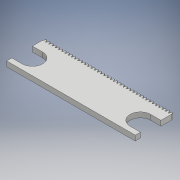
# Autodesk Inventor part: RescueKit-Slidev2
Saved by Autodesk Inventor 2018.3 (Build 223284000, 284)
## iProperties
Created: 2019-03-13
Part Number: RescueKit-Slidev2
Material: 一般
Document SubType Name: Modeling
Designer: shun2
Density: 1 g/cm^3
Appearance: 既定
Author: shun2
Autodesk Inventor part; units mm, degrees
ref_plane "YZ Plane" through (0, 0, 0) normal (1, 0, 0) x (0, 1, 0)
ref_plane "XZ Plane" through (0, 0, 0) normal (0, 1, 0) x (-1, 0, 0)
ref_plane "XY Plane" through (0, 0, 0) normal (0, 0, 1) x (1, 0, 0)
sketch "スケッチ1" plane through (0, 0, 0) normal (0, 0, 1) x (1, 0, 0)
  line L0 (125, 35.6665) -> (124.5146, 37)
  line L1 (124.5146, 37) -> (123.6718, 37)
  line L2 (123.6718, 37) -> (122.9438, 35)
  arc A0 (122.5868, 34.75) -> (122.9438, 35) centre (122.5868, 35.13) ccw
  line L3 (122.5868, 34.75) -> (122.458, 34.75)
  arc A1 (122.101, 35) -> (122.458, 34.75) centre (122.458, 35.13) ccw
  line L4 (122.101, 35) -> (121.373, 37)
  line L5 (121.373, 37) -> (120.5302, 37)
  line L6 (120.5302, 37) -> (119.8022, 35)
  arc A2 (119.4452, 34.75) -> (119.8022, 35) centre (119.4452, 35.13) ccw
  line L7 (119.4452, 34.75) -> (119.3164, 34.75)
  arc A3 (118.9594, 35) -> (119.3164, 34.75) centre (119.3164, 35.13) ccw
  line L8 (118.9594, 35) -> (118.2314, 37)
  line L9 (118.2314, 37) -> (117.3886, 37)
  line L10 (117.3886, 37) -> (116.6606, 35)
  arc A4 (116.3036, 34.75) -> (116.6606, 35) centre (116.3036, 35.13) ccw
  line L11 (116.3036, 34.75) -> (116.1748, 34.75)
  arc A5 (115.8178, 35) -> (116.1748, 34.75) centre (116.1748, 35.13) ccw
  line L12 (115.8178, 35) -> (115.0898, 37)
  line L13 (115.0898, 37) -> (114.247, 37)
  line L14 (114.247, 37) -> (113.519, 35)
  arc A6 (113.162, 34.75) -> (113.519, 35) centre (113.162, 35.13) ccw
  line L15 (113.162, 34.75) -> (113.0332, 34.75)
  arc A7 (112.6762, 35) -> (113.0332, 34.75) centre (113.0332, 35.13) ccw
  line L16 (112.6762, 35) -> (111.9482, 37)
  line L17 (111.9482, 37) -> (111.1054, 37)
  line L18 (111.1054, 37) -> (110.3774, 35)
  arc A8 (110.0204, 34.75) -> (110.3774, 35) centre (110.0204, 35.13) ccw
  line L19 (110.0204, 34.75) -> (109.8916, 34.75)
  arc A9 (109.5346, 35) -> (109.8916, 34.75) centre (109.8916, 35.13) ccw
  line L20 (109.5346, 35) -> (108.8066, 37)
  line L21 (108.8066, 37) -> (107.9638, 37)
  line L22 (107.9638, 37) -> (107.2358, 35)
  arc A10 (106.8788, 34.75) -> (107.2358, 35) centre (106.8788, 35.13) ccw
  line L23 (106.8788, 34.75) -> (106.75, 34.75)
  arc A11 (106.393, 35) -> (106.75, 34.75) centre (106.75, 35.13) ccw
  line L24 (106.393, 35) -> (105.665, 37)
  line L25 (105.665, 37) -> (104.8222, 37)
  line L26 (104.8222, 37) -> (104.0942, 35)
  arc A12 (103.7372, 34.75) -> (104.0942, 35) centre (103.7372, 35.13) ccw
  line L27 (103.7372, 34.75) -> (103.6084, 34.75)
  arc A13 (103.2514, 35) -> (103.6084, 34.75) centre (103.6084, 35.13) ccw
  line L28 (103.2514, 35) -> (102.5234, 37)
  line L29 (102.5234, 37) -> (101.6806, 37)
  line L30 (101.6806, 37) -> (100.9526, 35)
  arc A14 (100.5956, 34.75) -> (100.9526, 35) centre (100.5956, 35.13) ccw
  line L31 (100.5956, 34.75) -> (100.4668, 34.75)
  arc A15 (100.1098, 35) -> (100.4668, 34.75) centre (100.4668, 35.13) ccw
  line L32 (100.1098, 35) -> (99.3818, 37)
  line L33 (99.3818, 37) -> (98.539, 37)
  line L34 (98.539, 37) -> (97.811, 35)
  arc A16 (97.454, 34.75) -> (97.811, 35) centre (97.454, 35.13) ccw
  line L35 (97.454, 34.75) -> (97.3252, 34.75)
  arc A17 (96.9682, 35) -> (97.3252, 34.75) centre (97.3252, 35.13) ccw
  line L36 (96.9682, 35) -> (96.2402, 37)
  line L37 (96.2402, 37) -> (95.3974, 37)
  line L38 (95.3974, 37) -> (94.6694, 35)
  arc A18 (94.3124, 34.75) -> (94.6694, 35) centre (94.3124, 35.13) ccw
  line L39 (94.3124, 34.75) -> (94.1836, 34.75)
  arc A19 (93.8266, 35) -> (94.1836, 34.75) centre (94.1836, 35.13) ccw
  line L40 (93.8266, 35) -> (93.0986, 37)
  line L41 (93.0986, 37) -> (92.2558, 37)
  line L42 (92.2558, 37) -> (91.5278, 35)
  arc A20 (91.1708, 34.75) -> (91.5278, 35) centre (91.1708, 35.13) ccw
  line L43 (91.1708, 34.75) -> (91.042, 34.75)
  arc A21 (90.685, 35) -> (91.042, 34.75) centre (91.042, 35.13) ccw
  line L44 (90.685, 35) -> (89.957, 37)
  line L45 (89.957, 37) -> (89.1142, 37)
  line L46 (89.1142, 37) -> (88.3862, 35)
  arc A22 (88.0292, 34.75) -> (88.3862, 35) centre (88.0292, 35.13) ccw
  line L47 (88.0292, 34.75) -> (87.9004, 34.75)
  arc A23 (87.5434, 35) -> (87.9004, 34.75) centre (87.9004, 35.13) ccw
  line L48 (87.5434, 35) -> (86.8154, 37)
  line L49 (86.8154, 37) -> (85.9726, 37)
  line L50 (85.9726, 37) -> (85.2446, 35)
  arc A24 (84.8876, 34.75) -> (85.2446, 35) centre (84.8876, 35.13) ccw
  line L51 (84.8876, 34.75) -> (84.7588, 34.75)
  arc A25 (84.4018, 35) -> (84.7588, 34.75) centre (84.7588, 35.13) ccw
  line L52 (84.4018, 35) -> (83.6738, 37)
  line L53 (83.6738, 37) -> (82.831, 37)
  line L54 (82.831, 37) -> (82.103, 35)
  arc A26 (81.746, 34.75) -> (82.103, 35) centre (81.746, 35.13) ccw
  line L55 (81.746, 34.75) -> (81.6172, 34.75)
  arc A27 (81.2602, 35) -> (81.6172, 34.75) centre (81.6172, 35.13) ccw
  line L56 (81.2602, 35) -> (80.5322, 37)
  line L57 (80.5322, 37) -> (79.6894, 37)
  line L58 (79.6894, 37) -> (78.9614, 35)
  arc A28 (78.6044, 34.75) -> (78.9614, 35) centre (78.6044, 35.13) ccw
  line L59 (78.6044, 34.75) -> (78.4756, 34.75)
  arc A29 (78.1186, 35) -> (78.4756, 34.75) centre (78.4756, 35.13) ccw
  line L60 (78.1186, 35) -> (77.3906, 37)
  line L61 (77.3906, 37) -> (76.5478, 37)
  line L62 (76.5478, 37) -> (75.8198, 35)
  arc A30 (75.4628, 34.75) -> (75.8198, 35) centre (75.4628, 35.13) ccw
  line L63 (75.4628, 34.75) -> (75.334, 34.75)
  arc A31 (74.977, 35) -> (75.334, 34.75) centre (75.334, 35.13) ccw
  line L64 (74.977, 35) -> (74.249, 37)
  line L65 (74.249, 37) -> (73.4062, 37)
  line L66 (73.4062, 37) -> (72.6782, 35)
  arc A32 (72.3212, 34.75) -> (72.6782, 35) centre (72.3212, 35.13) ccw
  line L67 (72.3212, 34.75) -> (72.1924, 34.75)
  arc A33 (71.8354, 35) -> (72.1924, 34.75) centre (72.1924, 35.13) ccw
  line L68 (71.8354, 35) -> (71.1074, 37)
  line L69 (71.1074, 37) -> (70.2646, 37)
  line L70 (70.2646, 37) -> (69.5366, 35)
  arc A34 (69.1796, 34.75) -> (69.5366, 35) centre (69.1796, 35.13) ccw
  line L71 (69.1796, 34.75) -> (69.0508, 34.75)
  arc A35 (68.6938, 35) -> (69.0508, 34.75) centre (69.0508, 35.13) ccw
  line L72 (68.6938, 35) -> (67.9658, 37)
  line L73 (67.9658, 37) -> (67.123, 37)
  line L74 (67.123, 37) -> (66.395, 35)
  arc A36 (66.038, 34.75) -> (66.395, 35) centre (66.038, 35.13) ccw
  line L75 (66.038, 34.75) -> (65.9092, 34.75)
  arc A37 (65.5522, 35) -> (65.9092, 34.75) centre (65.9092, 35.13) ccw
  line L76 (65.5522, 35) -> (64.8242, 37)
  line L77 (64.8242, 37) -> (63.9814, 37)
  line L78 (63.9814, 37) -> (63.2534, 35)
  arc A38 (62.8964, 34.75) -> (63.2534, 35) centre (62.8964, 35.13) ccw
  line L79 (62.8964, 34.75) -> (62.7676, 34.75)
  arc A39 (62.4106, 35) -> (62.7676, 34.75) centre (62.7676, 35.13) ccw
  line L80 (62.4106, 35) -> (61.6826, 37)
  line L81 (61.6826, 37) -> (60.8398, 37)
  line L82 (60.8398, 37) -> (60.1118, 35)
  arc A40 (59.7548, 34.75) -> (60.1118, 35) centre (59.7548, 35.13) ccw
  line L83 (59.7548, 34.75) -> (59.626, 34.75)
  arc A41 (59.269, 35) -> (59.626, 34.75) centre (59.626, 35.13) ccw
  line L84 (59.269, 35) -> (58.541, 37)
  line L85 (58.541, 37) -> (57.6982, 37)
  line L86 (57.6982, 37) -> (56.9702, 35)
  arc A42 (56.6132, 34.75) -> (56.9702, 35) centre (56.6132, 35.13) ccw
  line L87 (56.6132, 34.75) -> (56.4844, 34.75)
  arc A43 (56.1274, 35) -> (56.4844, 34.75) centre (56.4844, 35.13) ccw
  line L88 (56.1274, 35) -> (55.3994, 37)
  line L89 (55.3994, 37) -> (54.5566, 37)
  line L90 (54.5566, 37) -> (53.8286, 35)
  arc A44 (53.4716, 34.75) -> (53.8286, 35) centre (53.4716, 35.13) ccw
  line L91 (53.4716, 34.75) -> (53.3428, 34.75)
  arc A45 (52.9858, 35) -> (53.3428, 34.75) centre (53.3428, 35.13) ccw
  line L92 (52.9858, 35) -> (52.2578, 37)
  line L93 (52.2578, 37) -> (51.415, 37)
  line L94 (51.415, 37) -> (50.687, 35)
  arc A46 (50.33, 34.75) -> (50.687, 35) centre (50.33, 35.13) ccw
  line L95 (50.33, 34.75) -> (50.2012, 34.75)
  arc A47 (49.8442, 35) -> (50.2012, 34.75) centre (50.2012, 35.13) ccw
  line L96 (49.8442, 35) -> (49.1162, 37)
  line L97 (49.1162, 37) -> (48.2734, 37)
  line L98 (48.2734, 37) -> (47.5454, 35)
  arc A48 (47.1884, 34.75) -> (47.5454, 35) centre (47.1884, 35.13) ccw
  line L99 (47.1884, 34.75) -> (47.0596, 34.75)
  arc A49 (46.7026, 35) -> (47.0596, 34.75) centre (47.0596, 35.13) ccw
  line L100 (46.7026, 35) -> (45.9746, 37)
  line L101 (45.9746, 37) -> (45.1318, 37)
  line L102 (45.1318, 37) -> (44.4038, 35)
  arc A50 (44.0468, 34.75) -> (44.4038, 35) centre (44.0468, 35.13) ccw
  line L103 (44.0468, 34.75) -> (43.918, 34.75)
  arc A51 (43.561, 35) -> (43.918, 34.75) centre (43.918, 35.13) ccw
  line L104 (43.561, 35) -> (42.833, 37)
  line L105 (42.833, 37) -> (41.9902, 37)
  line L106 (41.9902, 37) -> (41.2622, 35)
  arc A52 (40.9052, 34.75) -> (41.2622, 35) centre (40.9052, 35.13) ccw
  line L107 (40.9052, 34.75) -> (40.7764, 34.75)
  arc A53 (40.4194, 35) -> (40.7764, 34.75) centre (40.7764, 35.13) ccw
  line L108 (40.4194, 35) -> (39.6914, 37)
  line L109 (39.6914, 37) -> (38.8486, 37)
  line L110 (38.8486, 37) -> (38.1206, 35)
  arc A54 (37.7636, 34.75) -> (38.1206, 35) centre (37.7636, 35.13) ccw
  line L111 (37.7636, 34.75) -> (37.6348, 34.75)
  arc A55 (37.2778, 35) -> (37.6348, 34.75) centre (37.6348, 35.13) ccw
  line L112 (37.2778, 35) -> (36.5498, 37)
  line L113 (36.5498, 37) -> (35.707, 37)
  line L114 (35.707, 37) -> (34.979, 35)
  arc A56 (34.622, 34.75) -> (34.979, 35) centre (34.622, 35.13) ccw
  line L115 (34.622, 34.75) -> (34.4932, 34.75)
  arc A57 (34.1362, 35) -> (34.4932, 34.75) centre (34.4932, 35.13) ccw
  line L116 (34.1362, 35) -> (33.4082, 37)
  line L117 (33.4082, 37) -> (32.5654, 37)
  line L118 (32.5654, 37) -> (31.8374, 35)
  arc A58 (31.4804, 34.75) -> (31.8374, 35) centre (31.4804, 35.13) ccw
  line L119 (31.4804, 34.75) -> (31.3516, 34.75)
  arc A59 (30.9946, 35) -> (31.3516, 34.75) centre (31.3516, 35.13) ccw
  line L120 (30.9946, 35) -> (30.2666, 37)
  line L121 (30.2666, 37) -> (29.4238, 37)
  line L122 (29.4238, 37) -> (28.6958, 35)
  arc A60 (28.3388, 34.75) -> (28.6958, 35) centre (28.3388, 35.13) ccw
  line L123 (28.3388, 34.75) -> (28.21, 34.75)
  arc A61 (27.853, 35) -> (28.21, 34.75) centre (28.21, 35.13) ccw
  line L124 (27.853, 35) -> (27.125, 37)
  line L125 (27.125, 37) -> (26.2822, 37)
  line L126 (26.2822, 37) -> (25.5542, 35)
  arc A62 (25.1972, 34.75) -> (25.5542, 35) centre (25.1972, 35.13) ccw
  line L127 (25.1972, 34.75) -> (25.0684, 34.75)
  arc A63 (24.7114, 35) -> (25.0684, 34.75) centre (25.0684, 35.13) ccw
  line L128 (24.7114, 35) -> (23.9834, 37)
  line L129 (23.9834, 37) -> (23.1406, 37)
  line L130 (23.1406, 37) -> (22.4126, 35)
  arc A64 (22.0556, 34.75) -> (22.4126, 35) centre (22.0556, 35.13) ccw
  line L131 (22.0556, 34.75) -> (21.9268, 34.75)
  arc A65 (21.5698, 35) -> (21.9268, 34.75) centre (21.9268, 35.13) ccw
  line L132 (21.5698, 35) -> (20.8418, 37)
  line L133 (20.8418, 37) -> (19.999, 37)
  line L134 (19.999, 37) -> (19.271, 35)
  arc A66 (18.914, 34.75) -> (19.271, 35) centre (18.914, 35.13) ccw
  line L135 (18.914, 34.75) -> (18.7852, 34.75)
  arc A67 (18.4282, 35) -> (18.7852, 34.75) centre (18.7852, 35.13) ccw
  line L136 (18.4282, 35) -> (17.7002, 37)
  line L137 (17.7002, 37) -> (16.8574, 37)
  line L138 (16.8574, 37) -> (16.1294, 35)
  arc A68 (15.7724, 34.75) -> (16.1294, 35) centre (15.7724, 35.13) ccw
  line L139 (15.7724, 34.75) -> (15.6436, 34.75)
  arc A69 (15.2866, 35) -> (15.6436, 34.75) centre (15.6436, 35.13) ccw
  line L140 (15.2866, 35) -> (14.5586, 37)
  line L141 (14.5586, 37) -> (13.7158, 37)
  line L142 (13.7158, 37) -> (12.9878, 35)
  arc A70 (12.6308, 34.75) -> (12.9878, 35) centre (12.6308, 35.13) ccw
  line L143 (12.6308, 34.75) -> (12.502, 34.75)
  arc A71 (12.145, 35) -> (12.502, 34.75) centre (12.502, 35.13) ccw
  line L144 (12.145, 35) -> (11.417, 37)
  line L145 (11.417, 37) -> (10.5742, 37)
  line L146 (10.5742, 37) -> (9.8462, 35)
  arc A72 (9.4892, 34.75) -> (9.8462, 35) centre (9.4892, 35.13) ccw
  line L147 (9.4892, 34.75) -> (9.3604, 34.75)
  arc A73 (9.0034, 35) -> (9.3604, 34.75) centre (9.3604, 35.13) ccw
  line L148 (9.0034, 35) -> (8.2754, 37)
  line L149 (8.2754, 37) -> (7.4326, 37)
  line L150 (7.4326, 37) -> (6.7046, 35)
  arc A74 (6.3476, 34.75) -> (6.7046, 35) centre (6.3476, 35.13) ccw
  line L151 (6.3476, 34.75) -> (6.2188, 34.75)
  arc A75 (5.8618, 35) -> (6.2188, 34.75) centre (6.2188, 35.13) ccw
  line L152 (5.8618, 35) -> (5.1338, 37)
  line L153 (5.1338, 37) -> (4.291, 37)
  line L154 (4.291, 37) -> (3.563, 35)
  arc A76 (3.206, 34.75) -> (3.563, 35) centre (3.206, 35.13) ccw
  line L155 (3.206, 34.75) -> (3.0772, 34.75)
  arc A77 (2.7202, 35) -> (3.0772, 34.75) centre (3.0772, 35.13) ccw
  line L156 (2.7202, 35) -> (1.9922, 37)
  line L157 (1.9922, 37) -> (1.1494, 37)
  line L158 (1.1494, 37) -> (0.4214, 35)
  arc A78 (0.0644, 34.75) -> (0.4214, 35) centre (0.0644, 35.13) ccw
  line L159 (0.0644, 34.75) -> (0, 34.75)
  line L160 (0, 34.75) -> (0, 25)
  line L161 (125, 25) -> (125, 35.6665)
  line L162 (0, 0) -> (125, 0)
  arc A79 (10, 5) -> (10, 25) centre (10, 15) ccw
  arc A80 (115, 25) -> (115, 5) centre (115, 15) ccw
  line L163 (10, 25) -> (0, 25)
  line L164 (10, 5) -> (0, 5)
  line L165 (115, 25) -> (125, 25)
  line L166 (115, 5) -> (125, 5)
  line L167 (0, 5) -> (0, 0)
  line L168 (125, 0) -> (125, 5)
  line L169 (0, 25) -> (10, 25)
  line L170 (115, 25) -> (125, 25)
  dimension "d10" = 20
  dimension "d11" = 20
  dimension "d12" = 125
  dimension "d13" = 5
  dimension "d14" = 10
  dimension "d15" = 115
  constraints: 342 end point, 162 point on circle, 81 centre point, 4 point on line, 3 perpendicular, 2 tangent, 1 horizontal, 1 parallel
  measures "d10" diameter of A79
  measures "d11" diameter of A80
  measures "d12" distance between parallel lines of L168 L167
  measures "d13" distance of L164.end L162.start
  measures "d14" distance from line of A79.centre L167
  measures "d15" distance from line of L167 A80.centre
extrude "押し出し1" add sketch "スケッチ1" along normal blind 5
